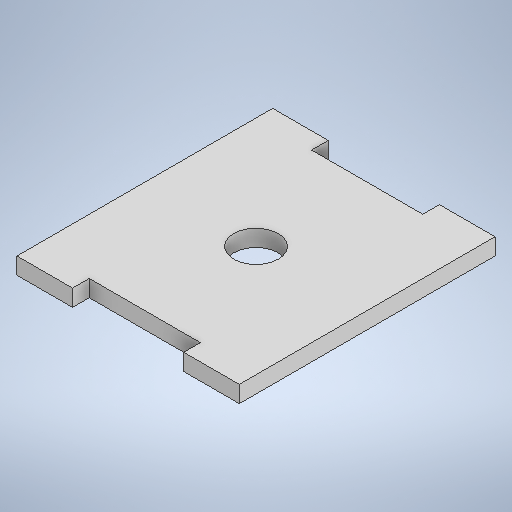
# Autodesk Inventor part: A_beam_end_mound_1
Saved by Autodesk Inventor 2025.2 (Build 292293000, 293)
## iProperties
Created: 2025-05-02
Part Number: A_beam_end_mound_1
Material: Generic
Document SubType Name: Sheet Metal
Designer: Caspe
Density: 1 g/cm^3
Sheet Metal Rule: Default_mm
Appearance: Default
Author: Caspe
Autodesk Inventor part; units mm, degrees
ref_plane "YZ Plane" through (0, 0, 0) normal (1, 0, 0) x (0, 1, 0)
ref_plane "XZ Plane" through (0, 0, 0) normal (0, 1, 0) x (-1, 0, 0)
ref_plane "XY Plane" through (0, 0, 0) normal (0, 0, 1) x (1, 0, 0)
sketch "Sketch1" plane through (0, 0, 0) normal (0, 1, 0) x (-1, 0, 0)
  line L0 (0, 0) -> (40, 0)
  line L1 (40, 0) -> (40, -40)
  line L2 (40, -40) -> (0, -40)
  line L3 (0, -40) -> (0, 0)
  line L4 (0, 0) -> (10, 0)
  line L5 (10, 0) -> (10, 3)
  line L6 (10, 3) -> (0, 3)
  line L7 (0, 3) -> (0, 0)
  line L8 (40, -20) -> (0, -20)
  line L9 (20, 0) -> (20, -40)
  line L10 (10, -40) -> (10, -43)
  line L11 (10, -43) -> (0, -43)
  line L12 (0, -43) -> (0, -40)
  line L13 (30, 0) -> (30, 3)
  line L14 (30, 3) -> (40, 3)
  line L15 (40, 3) -> (40, 0)
  line L16 (30, -40) -> (30, -43)
  line L17 (30, -43) -> (40, -43)
  line L18 (40, -43) -> (40, -40)
  circle A0 centre (20, -20) radius 4
  dimension "d0" = 40
  dimension "d1" = 40
  dimension "d2" = 10
  dimension "d3" = 3
  dimension "d5" = 8
  measures "d0" distance of L1.end L2.end
  measures "d1" distance of L0.end L1.end
  measures "d2" distance of L6.end L5.end
  measures "d3" distance of L5.end L4.end
  measures "d5" diameter of A0
extrude "Plate1" add sketch "Sketch1" along normal blind 3 contours L7 L6 L5 L0 | L0 L9 A0 L8 L3 | L8 A0 L9 L2 L3 | L0 L1 L8 A0 L9 | L2 L10 L11 L12 | L13 L14 L15 L0 | A0 L8 L1 L2 L9 | L2 L18 L17 L16
equation "\"d4\" = Thickness"
equation "\"BendRadius\" = Thickness"
equation "\"BendReliefWidth\" = Thickness"
equation "\"BendReliefDepth\" = 0.5 * Thickness"
equation "\"CornerReliefSize\" = 4 * Thickness"
equation "\"MinimumRemnant\" = 2 * Thickness"
equation "\"TransitionRadius\" = BendRadius"
equation "\"JacobiRadiusSize\" = BendRadius"
equation "\"GapSize\" = Thickness"
equation "\"Thickness\" = 3"
body "Solid1"
